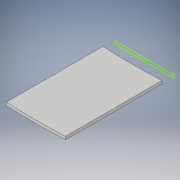
# Autodesk Inventor part: Board3.0
Saved by Autodesk Inventor 2019 (Build 230136000, 136)
## iProperties
Created: 2020-11-02
Part Number: Board3.0
Material: Generic
Document SubType Name: Modeling
Designer: Anass Hamdi
Density: 1 g/cm^3
Appearance: Default
Author: Anass Hamdi
Autodesk Inventor part; units mm, degrees
ref_plane "YZ Plane" through (0, 0, 0) normal (1, 0, 0) x (0, 1, 0)
ref_plane "XZ Plane" through (0, 0, 0) normal (0, 1, 0) x (-1, 0, 0)
ref_plane "XY Plane" through (0, 0, 0) normal (0, 0, 1) x (1, 0, 0)
sketch "Sketch3" plane through (0, 0, 0) normal (0, 0, 1) x (1, 0, 0)
  line L0 (101.1005, 5.849) -> (0, 7) construction
  line L1 (0, 7) -> (0, 3.3695) construction
  line L2 (101.7603, -4.151) -> (0, -4.151) construction
  line L3 (0, -4.151) -> (0, -6.6305) construction
  line L4 (101.7603, -4.151) -> (101.1005, 5.849)
  line L5 (-101.1005, 5.849) -> (0, 7) construction
  line L6 (-101.7603, -4.151) -> (0, -4.151) construction
  arc A0 (-101.7603, -4.151) -> (101.7603, -4.151) centre (0, 2082.8259) ccw
  arc A1 (-101.1005, 5.849) -> (101.1005, 5.849) centre (0, 2065.8348) ccw
  line L7 (-101.7603, -4.151) -> (-101.1005, 5.849)
  point P0 (0, 0)
  dimension "d24" = 10
  dimension "d78" = 10
  dimension "d80" = 10
  dimension "d81" = 101.1005
  dimension "d82" = 3.6305
  dimension "d83" = 0.6598
  dimension "d84" = 101.7603
  dimension "d85" = 2.4794
  constraints: 16 end point, 6 point on circle, 4 coincident, 2 centre point, 1 horizontal, 1 perpendicular, 1 vertical
  measures "d24" distance of L1.end L3.end
  measures "d78" vertical distance of L0.start L2.start
  measures "d80" distance of L3.end L1.end
  measures "d81" horizontal distance of L0.start L0.end
  measures "d82" distance of L0.end L1.end
  measures "d83" horizontal distance of L2.start L0.start
  measures "d84" distance of L2.start L2.end
  measures "d85" distance of L2.end L3.end
extrude "Extrusion2" add sketch "Sketch3" along normal mid plane 330
ref_plane "Work Plane27" through (101.1005, 5.849, 0) normal (0.9978305, 0.0658354, 0) x (0, 0, 1)
sketch "Sketch54" plane through (101.1005, 5.849, 0) normal (0.9978305, 0.0658354, 0) x (0, 0, 1)
  line L0 (-165, 10.0217) -> (-165, 0)
  line L1 (-165, 10.0217) -> (-336.45, 10.0217) construction
  line L2 (-336.45, 10.0217) -> (-336.45, -39.9783) construction
  point P0 (0, -0.8197)
  dimension "d162" = 171.45
  dimension "d163" = 50
  constraints: 6 end point, 2 vertical, 1 horizontal
  measures "d162" distance of L0.start L1.end
  measures "d163" distance of L1.end L2.end
sketch "Sketch56" plane through (101.1005, 5.849, 0) normal (0.9978305, 0.0658354, 0) x (0, 0, 1)
  line L0 (-165, 0) -> (-165, 10.0217)
  point P0 (0, -0.8197)
  constraints: 2 end point, 1 vertical
ref_plane "Work Plane28" through (0, 0, -205) normal (0, 0, -1) x (-1, 0, 0)
sketch "Sketch57" plane through (0, 0, -205) normal (0, 0, -1) x (-1, 0, 0)
  line L0 (0, 3.3695) -> (-101.1005, 3.3695)
  line L1 (0, -6.6305) -> (-101.7603, -6.6305)
  line L2 (-101.7603, -6.6305) -> (-101.1005, 3.3695)
  line L3 (0, 3.3695) -> (101.1005, 3.3695)
  line L4 (0, 3.3695) -> (101.1005, 3.3695) construction
  line L5 (0, -6.6305) -> (101.7603, -6.6305)
  line L6 (0, -6.6305) -> (101.7603, -6.6305) construction
  line L7 (101.7603, -6.6305) -> (101.1005, 3.3695)
  constraints: 16 end point, 2 collinear, 2 horizontal
sketch "Sketch61" plane through (101.1005, 5.849, 0) normal (0.9978305, 0.0658354, 0) x (0, 0, 1)
  point P0 (0, -0.8197)
  point P1 (-205, 2.474)
  point P2 (-205, 12.4958)
body "Solid2"
